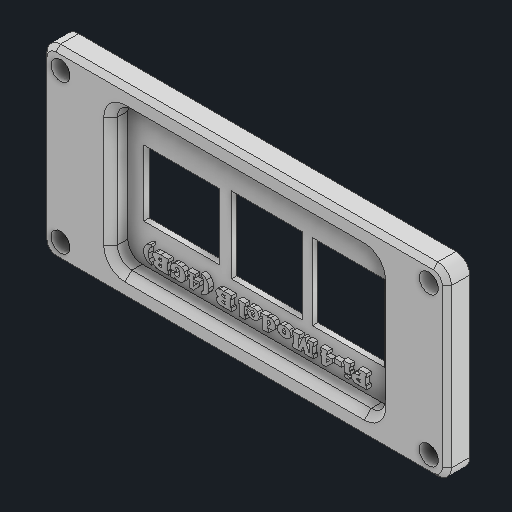
# Autodesk Inventor part: RaspberryPi_IO_Shield
Saved by Autodesk Inventor 2024 (Build 280153000, 153)
## iProperties
Created: 2025-09-25
Part Number: RaspberryPi_IO_Shield
Material: Generic
Document SubType Name: Modeling
Designer: kevin
Density: 1 g/cm^3
Appearance: Default
Author: kevin
Autodesk Inventor part; units mm, degrees
ref_plane "YZ Plane" through (0, 0, 0) normal (1, 0, 0) x (0, 1, 0)
ref_plane "XZ Plane" through (0, 0, 0) normal (0, 1, 0) x (-1, 0, 0)
ref_plane "XY Plane" through (0, 0, 0) normal (0, 0, 1) x (1, 0, 0)
sketch "Sketch1" plane through (0, 0, 0) normal (0, 0, 1) x (1, 0, 0)
  line L0 (56, 3) -> (56, -27.7344) construction
  line L1 (3, -24.7344) -> (53, -24.7344) construction
  line L2 (2.0246, -19.35) -> (2.0246, -4.85) projected
  line L3 (18.6077, -19.35) -> (2.0246, -19.35) projected
  line L4 (18.6077, -4.85) -> (18.6077, -19.35) projected
  line L5 (2.0246, -4.85) -> (18.6077, -4.85) projected
  line L6 (21.2876, -3.961) -> (36.872, -3.961) projected
  line L7 (21.2876, -20.7344) -> (21.2876, -3.961) projected
  line L8 (36.872, -20.7344) -> (21.2876, -20.7344) projected
  line L9 (36.872, -3.961) -> (36.872, -20.7344) projected
  line L10 (39.1307, -20.7344) -> (39.1307, -3.961) projected
  line L11 (54.9615, -20.7344) -> (39.1307, -20.7344) projected
  line L12 (54.9615, -3.961) -> (54.9615, -20.7344) projected
  line L13 (39.1307, -3.961) -> (54.9615, -3.961) projected
  line L14 (0, 3) -> (56, 3) projected
  line L15 (56, 0) -> (56, 3) projected
  line L16 (0, 0) -> (0, 3) projected
  line L17 (0, -27.7344) -> (0, 3) construction
  line L18 (56, -27.7344) -> (0, -27.7344) projected
  line L19 (3, -24.7344) -> (53, -24.7344) construction
  line L20 (57.5, 3) -> (57.5, -29.2344)
  line L21 (-1.5, -29.2344) -> (-1.5, 3)
  line L22 (56, -27.7344) -> (57.5, -27.7344)
  line L23 (0, -27.7344) -> (-1.5, -27.7344)
  line L24 (0, 3) -> (-1.5, 3)
  line L25 (56, 3) -> (57.5, 3)
  dimension "d0" = 1.5
  constraints: 12 end point, 3 point on line, 2 equal length, 1 perpendicular
  measures "d0" distance between parallel lines of L0 L20
extrude "Extrusion1" add sketch "Sketch1" along normal blind 1.2
sketch "Sketch2" plane through (0, 0, 1.2) normal (0, 0, 1) x (1, 0, 0)
  line L0 (54.9239, -26.0308) -> (0.076, -26.0308) construction
  line L1 (0.076, -26.0308) -> (0.076, -21.6275) construction
  line L2 (0.076, -21.6275) -> (54.9239, -21.6275) construction
  line L3 (54.9239, -21.6275) -> (54.9239, -26.0308) construction
  line L4 (50.2648, -22.9237) -> (52.0447, -22.9237)
  line L5 (52.0447, -22.9237) -> (52.0447, -23.6541)
  line L6 (52.0447, -23.6541) -> (51.7489, -23.6541)
  line L7 (51.7489, -23.6541) -> (51.7489, -25.2412)
  line L8 (51.7489, -25.2412) -> (52.0447, -25.2412)
  line L9 (52.0447, -25.2412) -> (52.0447, -25.9717)
  line L10 (52.0447, -25.9717) -> (50.1774, -25.9717)
  spline S0 degree 2 poles (50.1774, -25.9717) (49.5343, -25.9717) (49.2359, -25.8456) knots 0 0 0 1 1 1
  spline S1 degree 2 poles (49.2359, -25.8456) (48.9376, -25.7196) (48.7987, -25.501) knots 0 0 0 1 1 1
  spline S2 degree 2 poles (48.7987, -25.501) (48.6572, -25.2823) (48.6572, -25.02) knots 0 0 0 1 1 1
  spline S3 degree 2 poles (48.6572, -25.02) (48.6572, -24.6984) (48.8244, -24.485) knots 0 0 0 1 1 1
  spline S4 degree 2 poles (48.8244, -24.485) (48.989, -24.2715) (49.2642, -24.1763) knots 0 0 0 1 1 1
  spline S5 degree 2 poles (49.2642, -24.1763) (49.5343, -24.0811) (50.095, -24.0811) knots 0 0 0 1 1 1
  line L11 (50.095, -24.0811) -> (50.5709, -24.0811)
  line L12 (50.5709, -24.0811) -> (50.5709, -23.6541)
  line L13 (50.5709, -23.6541) -> (50.2648, -23.6541)
  line L14 (50.2648, -23.6541) -> (50.2648, -22.9237)
  line L15 (50.5709, -25.3029) -> (50.5709, -24.7319)
  line L16 (50.5709, -24.7319) -> (50.342, -24.7319)
  spline S6 degree 2 poles (50.342, -24.7319) (50.1002, -24.7319) (49.9922, -24.7885) knots 0 0 0 1 1 1
  spline S7 degree 2 poles (49.9922, -24.7885) (49.8867, -24.8451) (49.8867, -25.0097) knots 0 0 0 1 1 1
  spline S8 degree 2 poles (49.8867, -25.0097) (49.8867, -25.1177) (49.9433, -25.1897) knots 0 0 0 1 1 1
  spline S9 degree 2 poles (49.9433, -25.1897) (49.9973, -25.2643) (50.0899, -25.2823) knots 0 0 0 1 1 1
  spline S10 degree 2 poles (50.0899, -25.2823) (50.1774, -25.3029) (50.3883, -25.3029) knots 0 0 0 1 1 1
  line L17 (50.3883, -25.3029) -> (50.5709, -25.3029)
  line L18 (46.885, -22.9237) -> (48.3897, -22.9237)
  line L19 (48.3897, -22.9237) -> (48.3897, -23.5924)
  line L20 (48.3897, -23.5924) -> (48.1711, -23.5924)
  line L21 (48.1711, -23.5924) -> (48.1711, -24.3795)
  line L22 (48.1711, -24.3795) -> (48.3897, -24.3795)
  line L23 (48.3897, -24.3795) -> (48.3897, -25.0483)
  line L24 (48.3897, -25.0483) -> (47.0702, -25.0483)
  line L25 (47.0702, -25.0483) -> (47.0702, -23.5924)
  line L26 (47.0702, -23.5924) -> (46.885, -23.5924)
  line L27 (46.885, -23.5924) -> (46.885, -22.9237)
  spline S11 degree 2 poles (48.2637, -25.6476) (48.2637, -25.8199) (48.0862, -25.9254) knots 0 0 0 1 1 1
  spline S12 degree 2 poles (48.0862, -25.9254) (47.9113, -26.0308) (47.6515, -26.0308) knots 0 0 0 1 1 1
  spline S13 degree 2 poles (47.6515, -26.0308) (47.3866, -26.0308) (47.2245, -25.9228) knots 0 0 0 1 1 1
  spline S14 degree 2 poles (47.2245, -25.9228) (47.0651, -25.8096) (47.0651, -25.6501) knots 0 0 0 1 1 1
  spline S15 degree 2 poles (47.0651, -25.6501) (47.0651, -25.4778) (47.2322, -25.3775) knots 0 0 0 1 1 1
  spline S16 degree 2 poles (47.2322, -25.3775) (47.3994, -25.2746) (47.6566, -25.2746) knots 0 0 0 1 1 1
  spline S17 degree 2 poles (47.6566, -25.2746) (47.9164, -25.2746) (48.0913, -25.3698) knots 0 0 0 1 1 1
  spline S18 degree 2 poles (48.0913, -25.3698) (48.2637, -25.4598) (48.2637, -25.6476) knots 0 0 0 1 1 1
  line L28 (44.9405, -23.5127) -> (46.5043, -23.5127)
  line L29 (46.5043, -23.5127) -> (46.5043, -24.4567)
  line L30 (46.5043, -24.4567) -> (44.9405, -24.4567)
  line L31 (44.9405, -24.4567) -> (44.9405, -23.5127)
  line L32 (41.895, -22.9237) -> (43.4872, -22.9237)
  line L33 (43.4872, -22.9237) -> (43.4872, -23.541)
  line L34 (43.4872, -23.541) -> (43.1194, -23.541)
  line L35 (43.1194, -23.541) -> (43.1194, -23.9268)
  line L36 (43.1194, -23.9268) -> (44.4029, -23.9268)
  line L37 (44.4029, -23.9268) -> (44.5726, -24.5621)
  line L38 (44.5726, -24.5621) -> (43.1502, -26.0308)
  line L39 (43.1502, -26.0308) -> (42.2088, -26.0308)
  line L40 (42.2088, -26.0308) -> (42.2088, -24.4669)
  line L41 (42.2088, -24.4669) -> (41.895, -24.4669)
  line L42 (41.895, -24.4669) -> (41.895, -23.9268)
  line L43 (41.895, -23.9268) -> (42.2088, -23.9268)
  line L44 (42.2088, -23.9268) -> (42.2088, -23.541)
  line L45 (42.2088, -23.541) -> (41.895, -23.541)
  line L46 (41.895, -23.541) -> (41.895, -22.9237)
  line L47 (43.9425, -24.4669) -> (43.1194, -24.4669)
  line L48 (43.1194, -24.4669) -> (43.1194, -25.3003)
  line L49 (43.1194, -25.3003) -> (43.9425, -24.4669)
  line L50 (39.1325, -22.9237) -> (40.3132, -22.9237)
  line L51 (40.3132, -22.9237) -> (40.3132, -23.6541)
  line L52 (40.3132, -23.6541) -> (40.0791, -23.6541)
  line L53 (40.0791, -23.6541) -> (40.0791, -25.2412)
  line L54 (40.0791, -25.2412) -> (40.3209, -25.2412)
  line L55 (40.3209, -25.2412) -> (40.3209, -25.9717)
  line L56 (40.3209, -25.9717) -> (38.4844, -25.9717)
  line L57 (38.4844, -25.9717) -> (38.0342, -24.7936)
  line L58 (38.0342, -24.7936) -> (37.5738, -25.9717)
  line L59 (37.5738, -25.9717) -> (35.7476, -25.9717)
  line L60 (35.7476, -25.9717) -> (35.7476, -25.2412)
  line L61 (35.7476, -25.2412) -> (35.9868, -25.2412)
  line L62 (35.9868, -25.2412) -> (35.9868, -23.6541)
  line L63 (35.9868, -23.6541) -> (35.7399, -23.6541)
  line L64 (35.7399, -23.6541) -> (35.7399, -22.9237)
  line L65 (35.7399, -22.9237) -> (37.332, -22.9237)
  line L66 (37.332, -22.9237) -> (37.332, -23.6541)
  line L67 (37.332, -23.6541) -> (37.0877, -23.6541)
  line L68 (37.0877, -23.6541) -> (37.0877, -25.3543)
  line L69 (37.0877, -25.3543) -> (38.0085, -22.9237)
  line L70 (38.0085, -22.9237) -> (38.4638, -22.9237)
  line L71 (38.4638, -22.9237) -> (39.3743, -25.3338)
  line L72 (39.3743, -25.3338) -> (39.3743, -23.6541)
  line L73 (39.3743, -23.6541) -> (39.1325, -23.6541)
  line L74 (39.1325, -23.6541) -> (39.1325, -22.9237)
  spline S19 degree 2 poles (35.3643, -23.9962) (35.3643, -24.4669) (34.9708, -24.7885) knots 0 0 0 1 1 1
  spline S20 degree 2 poles (34.9708, -24.7885) (34.5747, -25.11) (33.9059, -25.11) knots 0 0 0 1 1 1
  spline S21 degree 2 poles (33.9059, -25.11) (33.232, -25.11) (32.8076, -24.7988) knots 0 0 0 1 1 1
  spline S22 degree 2 poles (32.8076, -24.7988) (32.3858, -24.4875) (32.3858, -23.9885) knots 0 0 0 1 1 1
  spline S23 degree 2 poles (32.3858, -23.9885) (32.3858, -23.505) (32.7896, -23.1834) knots 0 0 0 1 1 1
  spline S24 degree 2 poles (32.7896, -23.1834) (33.1909, -22.8619) (33.8519, -22.8619) knots 0 0 0 1 1 1
  spline S25 degree 2 poles (33.8519, -22.8619) (34.567, -22.8619) (34.9656, -23.1834) knots 0 0 0 1 1 1
  spline S26 degree 2 poles (34.9656, -23.1834) (35.3643, -23.505) (35.3643, -23.9962) knots 0 0 0 1 1 1
  spline S27 degree 2 poles (34.2506, -23.9937) (34.2506, -23.4844) (33.8853, -23.4844) knots 0 0 0 1 1 1
  spline S28 degree 2 poles (33.8853, -23.4844) (33.4995, -23.4844) (33.4995, -23.9962) knots 0 0 0 1 1 1
  spline S29 degree 2 poles (33.4995, -23.9962) (33.4995, -24.2303) (33.5947, -24.3615) knots 0 0 0 1 1 1
  spline S30 degree 2 poles (33.5947, -24.3615) (33.6899, -24.4901) (33.8673, -24.4901) knots 0 0 0 1 1 1
  spline S31 degree 2 poles (33.8673, -24.4901) (34.0397, -24.4901) (34.1451, -24.3641) knots 0 0 0 1 1 1
  spline S32 degree 2 poles (34.1451, -24.3641) (34.2506, -24.2355) (34.2506, -23.9937) knots 0 0 0 1 1 1
  line L75 (28.7539, -23.5924) -> (28.7539, -22.9237)
  line L76 (28.7539, -22.9237) -> (30.1326, -22.9237)
  line L77 (30.1326, -22.9237) -> (30.1326, -23.0651)
  spline S33 degree 2 poles (30.1326, -23.0651) (30.4387, -22.8851) (30.8399, -22.8851) knots 0 0 0 1 1 1
  spline S34 degree 2 poles (30.8399, -22.8851) (31.29, -22.8851) (31.6347, -23.1577) knots 0 0 0 1 1 1
  spline S35 degree 2 poles (31.6347, -23.1577) (31.982, -23.4329) (31.982, -23.9422) knots 0 0 0 1 1 1
  spline S36 degree 2 poles (31.982, -23.9422) (31.982, -24.4927) (31.663, -24.791) knots 0 0 0 1 1 1
  spline S37 degree 2 poles (31.663, -24.791) (31.3415, -25.0868) (30.8065, -25.0868) knots 0 0 0 1 1 1
  spline S38 degree 2 poles (30.8065, -25.0868) (30.4129, -25.0868) (30.1326, -24.9119) knots 0 0 0 1 1 1
  line L78 (30.1326, -24.9119) -> (30.1326, -25.3029)
  line L79 (30.1326, -25.3029) -> (30.4027, -25.3029)
  line L80 (30.4027, -25.3029) -> (30.4027, -25.9717)
  line L81 (30.4027, -25.9717) -> (29.0291, -25.9717)
  line L82 (29.0291, -25.9717) -> (29.0291, -23.5924)
  line L83 (29.0291, -23.5924) -> (28.7539, -23.5924)
  spline S39 degree 2 poles (30.1249, -23.9937) (30.1249, -24.1943) (30.2175, -24.3281) knots 0 0 0 1 1 1
  spline S40 degree 2 poles (30.2175, -24.3281) (30.3101, -24.4592) (30.4901, -24.4592) knots 0 0 0 1 1 1
  spline S41 degree 2 poles (30.4901, -24.4592) (30.8656, -24.4592) (30.8656, -23.9757) knots 0 0 0 1 1 1
  spline S42 degree 2 poles (30.8656, -23.9757) (30.8656, -23.775) (30.773, -23.6464) knots 0 0 0 1 1 1
  spline S43 degree 2 poles (30.773, -23.6464) (30.683, -23.5153) (30.5004, -23.5153) knots 0 0 0 1 1 1
  spline S44 degree 2 poles (30.5004, -23.5153) (30.3332, -23.5153) (30.2277, -23.631) knots 0 0 0 1 1 1
  spline S45 degree 2 poles (30.2277, -23.631) (30.1249, -23.7467) (30.1249, -23.9937) knots 0 0 0 1 1 1
  line L84 (26.6216, -23.595) -> (25.7136, -23.4844)
  spline S46 degree 2 poles (25.7136, -23.4844) (25.7728, -23.3403) (25.994, -23.1166) (26.1509, -23.0317) knots 0 0 0 1 2 2 2
  spline S47 degree 2 poles (26.1509, -23.0317) (26.4673, -22.8619) (26.9097, -22.8619) knots 0 0 0 1 1 1
  spline S48 degree 2 poles (26.9097, -22.8619) (27.653, -22.8619) (28.026, -23.1706) knots 0 0 0 1 1 1
  spline S49 degree 2 poles (28.026, -23.1706) (28.4015, -23.4767) (28.4015, -23.9757) knots 0 0 0 1 1 1
  spline S50 degree 2 poles (28.4015, -23.9757) (28.4015, -24.4618) (28.0311, -24.7859) knots 0 0 0 1 1 1
  spline S51 degree 2 poles (28.0311, -24.7859) (27.6659, -25.11) (27.0383, -25.11) knots 0 0 0 1 1 1
  spline S52 degree 2 poles (27.0383, -25.11) (26.4364, -25.11) (26.0583, -24.8039) knots 0 0 0 1 1 1
  spline S53 degree 2 poles (26.0583, -24.8039) (25.6853, -24.4978) (25.6622, -23.8754) knots 0 0 0 1 1 1
  line L85 (25.6622, -23.8754) -> (27.3341, -23.8754)
  spline S54 degree 2 poles (27.3341, -23.8754) (27.3289, -23.3583) (26.9508, -23.3583) knots 0 0 0 1 1 1
  spline S55 degree 2 poles (26.9508, -23.3583) (26.7219, -23.3583) (26.6216, -23.595) knots 0 0 0 1 1 1
  line L86 (27.3212, -24.1531) -> (26.7013, -24.1531)
  spline S56 degree 2 poles (26.7013, -24.1531) (26.6988, -24.22) (26.6988, -24.2277) knots 0 0 0 1 1 1
  spline S57 degree 2 poles (26.6988, -24.2277) (26.6988, -24.4001) (26.7862, -24.5158) knots 0 0 0 1 1 1
  spline S58 degree 2 poles (26.7862, -24.5158) (26.8737, -24.6264) (27.0177, -24.6264) knots 0 0 0 1 1 1
  spline S59 degree 2 poles (27.0177, -24.6264) (27.1669, -24.6264) (27.244, -24.503) knots 0 0 0 1 1 1
  spline S60 degree 2 poles (27.244, -24.503) (27.3238, -24.3795) (27.3238, -24.1969) knots 0 0 0 1 1 1
  spline S61 degree 2 poles (27.3238, -24.1969) (27.3238, -24.1737) (27.3212, -24.1531) knots 0 0 0 1 1 1
  line L87 (23.7922, -22.9237) -> (25.3149, -22.9237)
  line L88 (25.3149, -22.9237) -> (25.3149, -23.5924)
  line L89 (25.3149, -23.5924) -> (25.0886, -23.5924)
  line L90 (25.0886, -23.5924) -> (25.0886, -25.3029)
  line L91 (25.0886, -25.3029) -> (25.3149, -25.3029)
  line L92 (25.3149, -25.3029) -> (25.3149, -25.9717)
  line L93 (25.3149, -25.9717) -> (23.9877, -25.9717)
  line L94 (23.9877, -25.9717) -> (23.9877, -23.5924)
  line L95 (23.9877, -23.5924) -> (23.7922, -23.5924)
  line L96 (23.7922, -23.5924) -> (23.7922, -22.9237)
  line L97 (20.6002, -22.9237) -> (22.3235, -22.9237)
  line L98 (22.3235, -22.9237) -> (22.3235, -23.6541)
  line L99 (22.3235, -23.6541) -> (22.0586, -23.6541)
  line L100 (22.0586, -23.6541) -> (22.0586, -25.2412)
  line L101 (22.0586, -25.2412) -> (22.3235, -25.2412)
  line L102 (22.3235, -25.2412) -> (22.3235, -25.9717)
  line L103 (22.3235, -25.9717) -> (20.4613, -25.9717)
  spline S62 degree 2 poles (20.4613, -25.9717) (19.9134, -25.9717) (19.615, -25.9074) knots 0 0 0 1 1 1
  spline S63 degree 2 poles (19.615, -25.9074) (19.3192, -25.843) (19.1495, -25.6476) knots 0 0 0 1 1 1
  spline S64 degree 2 poles (19.1495, -25.6476) (18.9797, -25.4469) (18.9797, -25.182) knots 0 0 0 1 1 1
  spline S65 degree 2 poles (18.9797, -25.182) (18.9797, -24.9248) (19.1418, -24.7705) knots 0 0 0 1 1 1
  spline S66 degree 2 poles (19.1418, -24.7705) (19.3038, -24.6136) (19.5405, -24.5518) knots 0 0 0 1 1 1
  spline S67 degree 2 poles (19.5405, -24.5518) (19.2164, -24.4541) (19.044, -24.2535) knots 0 0 0 1 1 1
  spline S68 degree 2 poles (19.044, -24.2535) (18.8691, -24.0477) (18.8691, -23.7905) knots 0 0 0 1 1 1
  spline S69 degree 2 poles (18.8691, -23.7905) (18.8691, -23.4844) (19.0672, -23.2709) knots 0 0 0 1 1 1
  spline S70 degree 2 poles (19.0672, -23.2709) (19.2627, -23.0574) (19.6073, -22.9905) knots 0 0 0 1 1 1
  spline S71 degree 2 poles (19.6073, -22.9905) (19.9469, -22.9237) (20.6002, -22.9237) knots 0 0 0 1 1 1
  line L104 (20.8805, -24.1917) -> (20.8805, -23.5924)
  line L105 (20.8805, -23.5924) -> (20.6156, -23.5924)
  spline S72 degree 2 poles (20.6156, -23.5924) (20.361, -23.5924) (20.2504, -23.6593) knots 0 0 0 1 1 1
  spline S73 degree 2 poles (20.2504, -23.6593) (20.1398, -23.7236) (20.1398, -23.8908) knots 0 0 0 1 1 1
  spline S74 degree 2 poles (20.1398, -23.8908) (20.1398, -24.0451) (20.2375, -24.1197) knots 0 0 0 1 1 1
  spline S75 degree 2 poles (20.2375, -24.1197) (20.3378, -24.1917) (20.6182, -24.1917) knots 0 0 0 1 1 1
  line L106 (20.6182, -24.1917) -> (20.8805, -24.1917)
  line L107 (20.8805, -25.3029) -> (20.8805, -24.7473)
  line L108 (20.8805, -24.7473) -> (20.6182, -24.7473)
  spline S76 degree 2 poles (20.6182, -24.7473) (20.3533, -24.7473) (20.2709, -24.8245) knots 0 0 0 1 1 1
  spline S77 degree 2 poles (20.2709, -24.8245) (20.1912, -24.9016) (20.1912, -25.0251) knots 0 0 0 1 1 1
  spline S78 degree 2 poles (20.1912, -25.0251) (20.1912, -25.1331) (20.2632, -25.218) knots 0 0 0 1 1 1
  spline S79 degree 2 poles (20.2632, -25.218) (20.3378, -25.3029) (20.6619, -25.3029) knots 0 0 0 1 1 1
  line L109 (20.6619, -25.3029) -> (20.8805, -25.3029)
  line L110 (15.6899, -22.5584) -> (15.6899, -21.9874)
  spline S80 degree 2 poles (15.6899, -21.9874) (16.0192, -22.0594) (16.5928, -22.3758) (16.8474, -22.6279) knots 0 0 0 1 2 2 2
  spline S81 degree 2 poles (16.8474, -22.6279) (17.349, -23.1217) (17.349, -24.0091) knots 0 0 0 1 1 1
  spline S82 degree 2 poles (17.349, -24.0091) (17.349, -24.539) (17.1766, -24.9119) knots 0 0 0 1 1 1
  spline S83 degree 2 poles (17.1766, -24.9119) (17.0017, -25.29) (16.6133, -25.5935) knots 0 0 0 1 1 1
  spline S84 degree 2 poles (16.6133, -25.5935) (16.2249, -25.8945) (15.6899, -26.0308) knots 0 0 0 1 1 1
  line L111 (15.6899, -26.0308) -> (15.6899, -25.4572)
  spline S85 degree 2 poles (15.6899, -25.4572) (15.9086, -25.4006) (16.068, -25.1023) knots 0 0 0 1 1 1
  spline S86 degree 2 poles (16.068, -25.1023) (16.2327, -24.8039) (16.2327, -24.0657) knots 0 0 0 1 1 1
  spline S87 degree 2 poles (16.2327, -24.0657) (16.2327, -23.3506) (16.1092, -23.024) knots 0 0 0 1 1 1
  spline S88 degree 2 poles (16.1092, -23.024) (15.9832, -22.6999) (15.6899, -22.5584) knots 0 0 0 1 1 1
  line L112 (12.6934, -22.9237) -> (14.2855, -22.9237)
  line L113 (14.2855, -22.9237) -> (14.2855, -23.541)
  line L114 (14.2855, -23.541) -> (13.9177, -23.541)
  line L115 (13.9177, -23.541) -> (13.9177, -23.9268)
  line L116 (13.9177, -23.9268) -> (15.2012, -23.9268)
  line L117 (15.2012, -23.9268) -> (15.371, -24.5621)
  line L118 (15.371, -24.5621) -> (13.9486, -26.0308)
  line L119 (13.9486, -26.0308) -> (13.0072, -26.0308)
  line L120 (13.0072, -26.0308) -> (13.0072, -24.4669)
  line L121 (13.0072, -24.4669) -> (12.6934, -24.4669)
  line L122 (12.6934, -24.4669) -> (12.6934, -23.9268)
  line L123 (12.6934, -23.9268) -> (13.0072, -23.9268)
  line L124 (13.0072, -23.9268) -> (13.0072, -23.541)
  line L125 (13.0072, -23.541) -> (12.6934, -23.541)
  line L126 (12.6934, -23.541) -> (12.6934, -22.9237)
  line L127 (14.7408, -24.4669) -> (13.9177, -24.4669)
  line L128 (13.9177, -24.4669) -> (13.9177, -25.3003)
  line L129 (13.9177, -25.3003) -> (14.7408, -24.4669)
  line L130 (9.9232, -23.9731) -> (10.2344, -23.9731)
  line L131 (10.2344, -23.9731) -> (10.2344, -24.5518)
  line L132 (10.2344, -24.5518) -> (8.8712, -24.5518)
  spline S89 degree 2 poles (8.8712, -24.5518) (8.8712, -24.0528) (8.9406, -23.8085) knots 0 0 0 1 1 1
  spline S90 degree 2 poles (8.9406, -23.8085) (9.0101, -23.5744) (9.2261, -23.3326) knots 0 0 0 1 1 1
  spline S91 degree 2 poles (9.2261, -23.3326) (9.4396, -23.0934) (9.7406, -22.9854) knots 0 0 0 1 1 1
  spline S92 degree 2 poles (9.7406, -22.9854) (10.0441, -22.8748) (10.3887, -22.8748) knots 0 0 0 1 1 1
  spline S93 degree 2 poles (10.3887, -22.8748) (10.9032, -22.8748) (11.325, -23.0471) knots 0 0 0 1 1 1
  spline S94 degree 2 poles (11.325, -23.0471) (11.7468, -23.2117) (11.9783, -23.5976) knots 0 0 0 1 1 1
  spline S95 degree 2 poles (11.9783, -23.5976) (12.2098, -23.9757) (12.2098, -24.4464) knots 0 0 0 1 1 1
  spline S96 degree 2 poles (12.2098, -24.4464) (12.2098, -25.1589) (11.7417, -25.5935) knots 0 0 0 1 1 1
  spline S97 degree 2 poles (11.7417, -25.5935) (11.2761, -26.0308) (10.6022, -26.0308) knots 0 0 0 1 1 1
  spline S98 degree 2 poles (10.6022, -26.0308) (10.0389, -26.0308) (9.72, -25.7556) knots 0 0 0 1 1 1
  line L133 (9.72, -25.7556) -> (9.72, -25.9717)
  line L134 (9.72, -25.9717) -> (8.9843, -25.9717)
  line L135 (8.9843, -25.9717) -> (8.9843, -24.9042)
  line L136 (8.9843, -24.9042) -> (9.72, -24.9042)
  spline S99 degree 2 poles (9.72, -24.9042) (9.8151, -25.1023) (10.1238, -25.3029) (10.3296, -25.3029) knots 0 0 0 1 2 2 2
  spline S100 degree 2 poles (10.3296, -25.3029) (10.6177, -25.3029) (10.754, -25.1151) knots 0 0 0 1 1 1
  spline S101 degree 2 poles (10.754, -25.1151) (10.8877, -24.9274) (10.8877, -24.4232) knots 0 0 0 1 1 1
  spline S102 degree 2 poles (10.8877, -24.4232) (10.8877, -23.9217) (10.7488, -23.7442) knots 0 0 0 1 1 1
  spline S103 degree 2 poles (10.7488, -23.7442) (10.6048, -23.5615) (10.3347, -23.5615) knots 0 0 0 1 1 1
  spline S104 degree 2 poles (10.3347, -23.5615) (9.9232, -23.5615) (9.9232, -23.9731) knots 0 0 0 1 1 1
  line L137 (6.7208, -22.9237) -> (8.4442, -22.9237)
  line L138 (8.4442, -22.9237) -> (8.4442, -23.6541)
  line L139 (8.4442, -23.6541) -> (8.1793, -23.6541)
  line L140 (8.1793, -23.6541) -> (8.1793, -25.2412)
  line L141 (8.1793, -25.2412) -> (8.4442, -25.2412)
  line L142 (8.4442, -25.2412) -> (8.4442, -25.9717)
  line L143 (8.4442, -25.9717) -> (6.582, -25.9717)
  spline S105 degree 2 poles (6.582, -25.9717) (6.0341, -25.9717) (5.7357, -25.9074) knots 0 0 0 1 1 1
  spline S106 degree 2 poles (5.7357, -25.9074) (5.4399, -25.843) (5.2702, -25.6476) knots 0 0 0 1 1 1
  spline S107 degree 2 poles (5.2702, -25.6476) (5.1004, -25.4469) (5.1004, -25.182) knots 0 0 0 1 1 1
  spline S108 degree 2 poles (5.1004, -25.182) (5.1004, -24.9248) (5.2624, -24.7705) knots 0 0 0 1 1 1
  spline S109 degree 2 poles (5.2624, -24.7705) (5.4245, -24.6136) (5.6611, -24.5518) knots 0 0 0 1 1 1
  spline S110 degree 2 poles (5.6611, -24.5518) (5.337, -24.4541) (5.1647, -24.2535) knots 0 0 0 1 1 1
  spline S111 degree 2 poles (5.1647, -24.2535) (4.9898, -24.0477) (4.9898, -23.7905) knots 0 0 0 1 1 1
  spline S112 degree 2 poles (4.9898, -23.7905) (4.9898, -23.4844) (5.1878, -23.2709) knots 0 0 0 1 1 1
  spline S113 degree 2 poles (5.1878, -23.2709) (5.3833, -23.0574) (5.728, -22.9905) knots 0 0 0 1 1 1
  spline S114 degree 2 poles (5.728, -22.9905) (6.0675, -22.9237) (6.7208, -22.9237) knots 0 0 0 1 1 1
  line L144 (7.0012, -24.1917) -> (7.0012, -23.5924)
  line L145 (7.0012, -23.5924) -> (6.7363, -23.5924)
  spline S115 degree 2 poles (6.7363, -23.5924) (6.4816, -23.5924) (6.371, -23.6593) knots 0 0 0 1 1 1
  spline S116 degree 2 poles (6.371, -23.6593) (6.2604, -23.7236) (6.2604, -23.8908) knots 0 0 0 1 1 1
  spline S117 degree 2 poles (6.2604, -23.8908) (6.2604, -24.0451) (6.3582, -24.1197) knots 0 0 0 1 1 1
  spline S118 degree 2 poles (6.3582, -24.1197) (6.4585, -24.1917) (6.7389, -24.1917) knots 0 0 0 1 1 1
  line L146 (6.7389, -24.1917) -> (7.0012, -24.1917)
  line L147 (7.0012, -25.3029) -> (7.0012, -24.7473)
  line L148 (7.0012, -24.7473) -> (6.7389, -24.7473)
  spline S119 degree 2 poles (6.7389, -24.7473) (6.4739, -24.7473) (6.3916, -24.8245) knots 0 0 0 1 1 1
  spline S120 degree 2 poles (6.3916, -24.8245) (6.3119, -24.9016) (6.3119, -25.0251) knots 0 0 0 1 1 1
  spline S121 degree 2 poles (6.3119, -25.0251) (6.3119, -25.1331) (6.3839, -25.218) knots 0 0 0 1 1 1
  spline S122 degree 2 poles (6.3839, -25.218) (6.4585, -25.3029) (6.7826, -25.3029) knots 0 0 0 1 1 1
  line L149 (6.7826, -25.3029) -> (7.0012, -25.3029)
  line L150 (4.6348, -25.4572) -> (4.6348, -26.0308)
  spline S123 degree 2 poles (4.6348, -26.0308) (3.9789, -25.8919) (3.4748, -25.3929) knots 0 0 0 1 1 1
  spline S124 degree 2 poles (3.4748, -25.3929) (2.9758, -24.8991) (2.9758, -24.0065) knots 0 0 0 1 1 1
  spline S125 degree 2 poles (2.9758, -24.0065) (2.9758, -23.4767) (3.1533, -23.0986) knots 0 0 0 1 1 1
  spline S126 degree 2 poles (3.1533, -23.0986) (3.3308, -22.7179) (3.7243, -22.4169) knots 0 0 0 1 1 1
  spline S127 degree 2 poles (3.7243, -22.4169) (4.123, -22.1134) (4.6348, -21.9874) knots 0 0 0 1 1 1
  line L151 (4.6348, -21.9874) -> (4.6348, -22.5584)
  spline S128 degree 2 poles (4.6348, -22.5584) (4.4188, -22.6176) (4.2567, -22.9185) knots 0 0 0 1 1 1
  spline S129 degree 2 poles (4.2567, -22.9185) (4.0921, -23.2169) (4.0921, -23.9525) knots 0 0 0 1 1 1
  spline S130 degree 2 poles (4.0921, -23.9525) (4.0921, -24.6701) (4.2156, -24.9942) knots 0 0 0 1 1 1
  spline S131 degree 2 poles (4.2156, -24.9942) (4.339, -25.3158) (4.6348, -25.4572) knots 0 0 0 1 1 1
  point P0 (0, 0)
  constraints: 2 other
extrude "Extrusion2" add sketch "Sketch2" along normal blind 1
fillet "Fillet1" radius 3.175 4 edges at (57.5, -27.7344, 0.6) (-1.5, -27.7344, 0.6) (-1.5, 3, 0.6) (57.5, 3, 0.6)
sketch "Sketch3" plane through (0, 0, 0) normal (0, 0, -1) x (-1, 0, 0)
  arc A0 (-54.325, 3) -> (-57.5, -0.175) centre (-54.325, -0.175) ccw projected
  line L0 (-57.5, -24.5594) -> (-57.5, -0.175) projected
  arc A1 (-57.5, -24.5594) -> (-54.325, -27.7344) centre (-54.325, -24.5594) ccw projected
  line L1 (-1.675, -27.7344) -> (-54.325, -27.7344) projected
  arc A2 (-1.675, -27.7344) -> (1.5, -24.5594) centre (-1.675, -24.5594) ccw projected
  line L2 (1.5, -0.175) -> (1.5, -24.5594) projected
  arc A3 (1.5, -0.175) -> (-1.675, 3) centre (-1.675, -0.175) ccw projected
  line L3 (-54.325, 3) -> (-1.675, 3) projected
  line L4 (-2.0246, -19.35) -> (-2.0246, -4.85) projected
  line L5 (-18.6077, -19.35) -> (-2.0246, -19.35) projected
  line L6 (-18.6077, -4.85) -> (-18.6077, -19.35) projected
  line L7 (-2.0246, -4.85) -> (-18.6077, -4.85) projected
  line L8 (-21.2876, -3.961) -> (-36.872, -3.961) projected
  line L9 (-21.2876, -20.7344) -> (-21.2876, -3.961) projected
  line L10 (-36.872, -20.7344) -> (-21.2876, -20.7344) projected
  line L11 (-36.872, -3.961) -> (-36.872, -20.7344) projected
  line L12 (-39.1307, -20.7344) -> (-39.1307, -3.961) projected
  line L13 (-54.9615, -20.7344) -> (-39.1307, -20.7344) projected
  line L14 (-54.9615, -3.961) -> (-54.9615, -20.7344) projected
  line L15 (-39.1307, -3.961) -> (-54.9615, -3.961) projected
  line L16 (-62.5, -24.5594) -> (-62.5, -0.175)
  line L17 (-69.5, 8) -> (13.5, 8)
  line L18 (6.5, -0.175) -> (6.5, -24.5594)
  line L19 (13.5, -32.7344) -> (-69.5, -32.7344)
  line L20 (-72.5, -29.7344) -> (-72.5, 5)
  line L21 (16.5, 5) -> (16.5, -29.7344)
  arc A4 (-72.5, -29.7344) -> (-69.5, -32.7344) centre (-69.5, -29.7344) ccw
  arc A5 (13.5, -32.7344) -> (16.5, -29.7344) centre (13.5, -29.7344) ccw
  arc A6 (16.5, 5) -> (13.5, 8) centre (13.5, 5) ccw
  arc A7 (-69.5, 8) -> (-72.5, 5) centre (-69.5, 5) ccw
  circle A8 centre (-68.5, -28.7344) radius 2.1
  circle A9 centre (12.5, -28.7344) radius 2.1
  circle A10 centre (12.5, 4) radius 2.1
  circle A11 centre (-68.5, 4) radius 2.1
  point P0 (0, 0)
  point P1 (-72.5, 8)
  point P2 (16.5, -32.7344)
  point P3 (-72.5, -32.7344)
  point P4 (16.5, 8)
  dimension "d6" = 5
  dimension "d7" = 15
  dimension "d10" = 15
  dimension "d14" = 3
  dimension "d15" = 4.2
  dimension "d16" = 4.2
  dimension "d17" = 4.2
  dimension "d18" = 4.2
  dimension "d19" = 4
  dimension "d20" = 4
  dimension "d21" = 4
  dimension "d22" = 4
  dimension "d23" = 4
  dimension "d24" = 4
  dimension "d25" = 4
  dimension "d26" = 4
  constraints: 12 end point, 8 centre point, 8 point on circle, 8 point on line, 8 tangent, 3 equal radius
  measures "d6" distance between parallel lines of L1 L19
  measures "d7" distance between parallel lines of L2 L21
  measures "d10" distance between parallel lines of L20 L0
  measures "d14" radius of A4
  measures "d15" diameter of A8
  measures "d16" diameter of A11
  measures "d17" diameter of A10
  measures "d18" diameter of A9
  measures "d19" distance from line of L19 A8.centre
  measures "d20" distance from line of L20 A8.centre
  measures "d21" distance from line of L20 A11.centre
  measures "d22" distance from line of L17 A11.centre
  measures "d23" distance from line of L21 A10.centre
  measures "d24" distance from line of L17 A10.centre
  measures "d25" distance from line of L21 A9.centre
  measures "d26" distance from line of L19 A9.centre
extrude "Extrusion3" add sketch "Sketch3" against normal blind 5 contours L17 A6 L21 A5 L19 A4 L20 A7
chamfer "Chamfer1" distance 1.5 angle 45 8 edges at (57.5, -12.3672, 5) (56.5701, -26.8045, 5) (28, -27.7344, 5) (-0.5701, -26.8045, 5) (-1.5, -12.3672, 5) (-0.5701, 2.0701, 5) (28, 3, 5) (56.5701, 2.0701, 5)
chamfer "Chamfer2" distance 1 angle 45 8 edges at (72.5, -12.3672, 5) (71.6213, 7.1213, 5) (28, 8, 5) (-15.6213, 7.1213, 5) (-16.5, -12.3672, 5) (-15.6213, -31.8557, 5) (28, -32.7344, 5) (71.6213, -31.8557, 5)
sketch "Sketch4" plane through (0, 0, 0) normal (0, 0, -1) x (-1, 0, 0)
  circle A0 centre (-68.5, -28.7344) radius 2.1 projected
  circle A1 centre (12.5, -28.7344) radius 2.1 projected
  circle A2 centre (12.5, 4) radius 2.1 projected
  circle A3 centre (-68.5, 4) radius 2.1 projected
  line L0 (-69.5, -32.7344) -> (13.5, -32.7344) projected
  arc A4 (13.5, -32.7344) -> (16.5, -29.7344) centre (13.5, -29.7344) ccw projected
  line L1 (16.5, -29.7344) -> (16.5, 5) projected
  arc A5 (16.5, 5) -> (13.5, 8) centre (13.5, 5) ccw projected
  line L2 (13.5, 8) -> (-69.5, 8) projected
  arc A6 (-69.5, 8) -> (-72.5, 5) centre (-69.5, 5) ccw projected
  line L3 (-72.5, 5) -> (-72.5, -29.7344) projected
  arc A7 (-72.5, -29.7344) -> (-69.5, -32.7344) centre (-69.5, -29.7344) ccw projected
  line L4 (-2.0246, -19.35) -> (-2.0246, -4.85) projected
  line L5 (-18.6077, -19.35) -> (-2.0246, -19.35) projected
  line L6 (-18.6077, -4.85) -> (-18.6077, -19.35) projected
  line L7 (-2.0246, -4.85) -> (-18.6077, -4.85) projected
  line L8 (-21.2876, -3.961) -> (-36.872, -3.961) projected
  line L9 (-21.2876, -20.7344) -> (-21.2876, -3.961) projected
  line L10 (-36.872, -20.7344) -> (-21.2876, -20.7344) projected
  line L11 (-36.872, -3.961) -> (-36.872, -20.7344) projected
  line L12 (-39.1307, -20.7344) -> (-39.1307, -3.961) projected
  line L13 (-54.9615, -20.7344) -> (-39.1307, -20.7344) projected
  line L14 (-54.9615, -3.961) -> (-54.9615, -20.7344) projected
  line L15 (-39.1307, -3.961) -> (-54.9615, -3.961) projected
  line L16 (0, 0) -> (0, 2) projected
  line L17 (-56, 0) -> (-56, 2) projected
  line L18 (4, 8) -> (4, -32.7344) construction
  line L19 (-28, -32.7344) -> (-28.0311, -24.7859) construction
  circle A8 centre (4, -15.7344) radius 1.6
  circle A9 centre (4, -4) radius 1.6
  circle A10 centre (-60.1322, -15.9855) radius 1.6
  circle A11 centre (-60.2241, -4.2515) radius 1.6
  dimension "d31" = 3.2
  dimension "d32" = 3.2
  dimension "d33" = 17
  dimension "d34" = 12
  constraints: 4 centre point, 4 end point, 4 point on line, 2 symmetric about line, 1 midpoint, 1 perpendicular, 2 other
  measures "d31" diameter of A8
  measures "d32" diameter of A9
  measures "d33" distance from line of L0 A8.centre
  measures "d34" distance from line of L2 A9.centre
extrude "Extrusion4" cut sketch "Sketch4" against normal blind 3 contours A8 | A9 | A10 | A11
equation "\"d16\" = d15"
equation "\"d17\" = d16"
equation "\"d18\" = d17"
equation "\"d20\" = d19"
equation "\"d21\" = d20"
equation "\"d22\" = d19"
equation "\"d23\" = d20"
equation "\"d24\" = d23"
equation "\"d25\" = d23"
equation "\"d26\" = d25"
equation "\"d32\" = d31"
body "Solid1"
